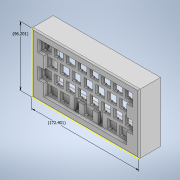
# Autodesk Inventor part: 1by2
Saved by Autodesk Inventor 2021 (Build 250183000, 183)
## iProperties
Created: 2021-06-14
Part Number: 1by2
Material: Generic
Document SubType Name: Modeling
Designer: UpahU
Density: 1 g/cm^3
Appearance: Default
Author: UpahU
Autodesk Inventor part; units mm, degrees
ref_plane "YZ Plane" through (0, 0, 0) normal (1, 0, 0) x (0, 1, 0)
ref_plane "XZ Plane" through (0, 0, 0) normal (0, 1, 0) x (-1, 0, 0)
ref_plane "XY Plane" through (0, 0, 0) normal (0, 0, 1) x (1, 0, 0)
sketch "Sketch1" plane through (0, 0, 0) normal (0, 0, 1) x (1, 0, 0)
  line L0 (0.0951, 96.5659) -> (172.496, 96.5659)
  line L1 (172.496, 96.5659) -> (172.496, 0.3652)
  line L2 (172.496, 0.3652) -> (0.0951, 0.3652)
  line L3 (0.0951, 0.3652) -> (0.0951, 96.5659)
  line L4 (136.445, 26.8911) -> (150.445, 26.8911)
  line L5 (150.445, 26.8911) -> (150.445, 12.8916)
  line L6 (150.445, 12.8916) -> (136.445, 12.8916)
  line L7 (136.445, 12.8916) -> (136.445, 26.8911)
  line L8 (117.394, 26.8911) -> (131.393, 26.8911)
  line L9 (131.3935, 26.8906) -> (131.393, 12.8911)
  line L10 (131.393, 12.8916) -> (117.394, 12.8916)
  line L11 (117.394, 12.8916) -> (117.394, 26.8911)
  line L12 (41.1939, 26.8911) -> (55.1931, 26.8911)
  line L13 (55.1931, 26.8911) -> (55.1931, 12.8916)
  line L14 (55.1931, 12.8916) -> (41.1939, 12.8916)
  line L15 (41.1939, 12.8916) -> (41.1939, 26.8911)
  line L16 (22.1437, 26.8911) -> (36.1446, 26.8911)
  line L17 (36.1446, 26.8911) -> (36.1446, 12.8916)
  line L18 (36.1446, 12.8916) -> (22.1437, 12.8916)
  line L19 (22.1437, 12.8916) -> (22.1437, 26.8911)
  line L20 (145.97, 45.9412) -> (159.97, 45.9412)
  line L21 (159.97, 45.9412) -> (159.97, 31.9416)
  line L22 (159.97, 31.9416) -> (145.97, 31.9416)
  line L23 (145.97, 31.9416) -> (145.97, 45.9412)
  line L24 (126.92, 45.9412) -> (140.92, 45.9412)
  line L25 (140.92, 45.9412) -> (140.92, 31.9416)
  line L26 (140.92, 31.9416) -> (126.92, 31.9416)
  line L27 (126.92, 31.9416) -> (126.92, 45.9412)
  line L28 (107.869, 45.9412) -> (121.868, 45.9412)
  line L29 (121.868, 45.9412) -> (121.868, 31.9416)
  line L30 (121.868, 31.9416) -> (107.869, 31.9416)
  line L31 (107.869, 31.9416) -> (107.869, 45.9412)
  line L32 (88.8199, 45.9412) -> (102.82, 45.9412)
  line L33 (102.82, 45.9412) -> (102.82, 31.9416)
  line L34 (102.82, 31.9416) -> (88.8199, 31.9416)
  line L35 (88.8199, 31.9416) -> (88.8199, 45.9412)
  line L36 (69.7699, 45.9412) -> (83.7696, 45.9412)
  line L37 (83.7696, 45.9412) -> (83.7696, 31.9416)
  line L38 (83.7696, 31.9416) -> (69.7699, 31.9416)
  line L39 (69.7699, 31.9416) -> (69.7699, 45.9412)
  line L40 (50.7199, 45.9412) -> (64.7196, 45.9412)
  line L41 (64.7196, 45.9412) -> (64.7196, 31.9416)
  line L42 (64.7196, 31.9416) -> (50.7199, 31.9416)
  line L43 (50.7199, 31.9416) -> (50.7199, 45.9412)
  line L44 (31.6701, 45.9412) -> (45.6696, 45.9412)
  line L45 (45.6696, 45.9412) -> (45.6696, 31.9416)
  line L46 (45.6696, 31.9416) -> (31.6701, 31.9416)
  line L47 (31.6701, 31.9416) -> (31.6701, 45.9412)
  line L48 (12.6201, 45.9412) -> (26.6196, 45.9412)
  line L49 (26.6196, 45.9412) -> (26.6196, 31.9416)
  line L50 (26.6196, 31.9416) -> (12.6201, 31.9416)
  line L51 (12.6201, 31.9416) -> (12.6201, 45.9412)
  line L52 (136.445, 64.9912) -> (150.445, 64.9912)
  line L53 (150.445, 64.9912) -> (150.445, 50.9916)
  line L54 (150.445, 50.9916) -> (136.445, 50.9916)
  line L55 (136.445, 50.9916) -> (136.445, 64.9912)
  line L56 (117.394, 64.9912) -> (131.393, 64.9912)
  line L57 (131.393, 64.9912) -> (131.393, 50.9916)
  line L58 (131.393, 50.9916) -> (117.394, 50.9916)
  line L59 (117.394, 50.9916) -> (117.394, 64.9912)
  line L60 (98.3439, 64.9912) -> (112.343, 64.9912)
  line L61 (112.343, 64.9912) -> (112.343, 50.9916)
  line L62 (112.343, 50.9916) -> (98.3439, 50.9916)
  line L63 (98.3439, 50.9916) -> (98.3439, 64.9912)
  line L64 (79.2939, 64.9912) -> (93.2931, 64.9912)
  line L65 (93.2931, 64.9912) -> (93.2931, 50.9916)
  line L66 (93.2931, 50.9916) -> (79.2939, 50.9916)
  line L67 (79.2939, 50.9916) -> (79.2939, 64.9912)
  line L68 (60.2439, 64.9912) -> (74.2431, 64.9912)
  line L69 (74.2431, 64.9912) -> (74.2431, 50.9916)
  line L70 (74.2431, 50.9916) -> (60.2439, 50.9916)
  line L71 (60.2439, 50.9916) -> (60.2439, 64.9912)
  line L72 (41.1939, 64.9912) -> (55.1931, 64.9912)
  line L73 (55.1931, 64.9912) -> (55.1931, 50.9916)
  line L74 (55.1931, 50.9916) -> (41.1939, 50.9916)
  line L75 (41.1939, 50.9916) -> (41.1939, 64.9912)
  line L76 (22.1437, 64.9912) -> (36.1446, 64.9912)
  line L77 (36.1446, 64.9912) -> (36.1446, 50.9916)
  line L78 (36.1446, 50.9916) -> (22.1437, 50.9916)
  line L79 (22.1437, 50.9916) -> (22.1437, 64.9912)
  line L80 (145.97, 84.0412) -> (159.97, 84.0412)
  line L81 (159.97, 84.0412) -> (159.97, 70.0416)
  line L82 (159.97, 70.0416) -> (145.97, 70.0416)
  line L83 (145.97, 70.0416) -> (145.97, 84.0412)
  line L84 (126.92, 84.0412) -> (140.92, 84.0412)
  line L85 (140.92, 84.0412) -> (140.92, 70.0416)
  line L86 (140.92, 70.0416) -> (126.92, 70.0416)
  line L87 (126.92, 70.0416) -> (126.92, 84.0412)
  line L88 (107.869, 84.0412) -> (121.868, 84.0412)
  line L89 (121.868, 84.0412) -> (121.868, 70.0416)
  line L90 (121.868, 70.0416) -> (107.869, 70.0416)
  line L91 (107.869, 70.0416) -> (107.869, 84.0412)
  line L92 (88.8199, 84.0412) -> (102.82, 84.0412)
  line L93 (102.82, 84.0412) -> (102.82, 70.0416)
  line L94 (102.82, 70.0416) -> (88.8199, 70.0416)
  line L95 (88.8199, 70.0416) -> (88.8199, 84.0412)
  line L96 (69.7699, 84.0412) -> (83.7696, 84.0412)
  line L97 (83.7696, 84.0412) -> (83.7696, 70.0416)
  line L98 (83.7696, 70.0416) -> (69.7699, 70.0416)
  line L99 (69.7699, 70.0416) -> (69.7699, 84.0412)
  line L100 (50.7199, 84.0412) -> (64.7196, 84.0412)
  line L101 (64.7196, 84.0412) -> (64.7196, 70.0416)
  line L102 (64.7196, 70.0416) -> (50.7199, 70.0416)
  line L103 (50.7199, 70.0416) -> (50.7199, 84.0412)
  line L104 (31.6701, 84.0412) -> (45.6696, 84.0412)
  line L105 (45.6696, 84.0412) -> (45.6696, 70.0416)
  line L106 (45.6696, 70.0416) -> (31.6701, 70.0416)
  line L107 (31.6701, 70.0416) -> (31.6701, 84.0412)
  line L108 (12.6201, 84.0412) -> (26.6196, 84.0412)
  line L109 (26.6196, 84.0412) -> (26.6196, 70.0416)
  line L110 (26.6196, 70.0416) -> (12.6201, 70.0416)
  line L111 (12.6201, 70.0416) -> (12.6201, 84.0412)
  line L112 (79.2923, 12.8885) -> (93.2923, 12.8885)
  line L113 (79.2923, 26.6885) -> (79.2923, 12.8885)
  line L114 (93.2923, 12.8885) -> (93.2923, 26.6885)
  arc A0 (108.8423, 29.7885) -> (108.3423, 30.2885) centre (108.3423, 29.7885) ccw
  arc A1 (101.8423, 10.6385) -> (102.3423, 10.1385) centre (102.3423, 10.6385) ccw
  arc A2 (108.3423, 10.1385) -> (108.8423, 10.6385) centre (108.3423, 10.6385) ccw
  line L115 (108.3423, 30.2885) -> (104.8423, 30.2885)
  line L116 (104.8423, 30.2885) -> (102.3423, 30.2885)
  line L117 (102.3423, 10.1385) -> (108.3423, 10.1385)
  line L118 (101.8423, 26.6885) -> (101.8423, 10.6385)
  line L119 (108.8423, 10.6385) -> (108.8423, 29.7885)
  arc A3 (64.2423, 30.2885) -> (63.7423, 29.7885) centre (64.2423, 29.7885) ccw
  arc A4 (63.7423, 10.6385) -> (64.2423, 10.1385) centre (64.2423, 10.6385) ccw
  arc A5 (70.2423, 10.1385) -> (70.7423, 10.6385) centre (70.2423, 10.6385) ccw
  line L120 (70.2423, 30.2885) -> (67.7423, 30.2885)
  line L121 (67.7423, 30.2885) -> (64.2423, 30.2885)
  line L122 (64.2423, 10.1385) -> (70.2423, 10.1385)
  line L123 (63.7423, 29.7885) -> (63.7423, 10.6385)
  line L124 (70.7423, 10.6385) -> (70.7423, 26.6885)
  line L125 (102.3423, 30.2885) -> (70.2423, 30.2885)
  line L126 (70.7423, 26.6885) -> (79.2923, 26.6885)
  line L127 (93.2923, 26.6885) -> (101.8423, 26.6885)
  point P0 (0.0951, 0.3652)
  point P1 (172.496, 0.3652)
  point P2 (131.3935, 26.8911)
  point P3 (131.393, 12.8916)
  point P4 (70.7423, 10.6385)
  point P5 (70.2423, 10.1385)
  point P6 (64.2423, 10.1385)
  point P7 (63.7423, 10.6385)
  point P8 (63.7423, 29.7885)
  point P9 (64.2423, 30.2885)
  point P10 (108.3423, 30.2885)
  point P11 (108.8423, 29.7885)
  point P12 (108.8423, 10.6385)
  point P13 (108.3423, 10.1385)
  point P14 (102.3423, 10.1385)
  point P15 (101.8423, 10.6385)
  point P16 (86.2923, 19.8914)
  constraints: 256 end point, 12 point on circle, 6 centre point
extrude "Extrusion1" add sketch "Sketch1" along normal blind 1.5
sketch "Sketch2" plane through (0, 0, 1.5) normal (0, 0, 1) x (1, 0, 0)
  line L0 (0.0951, 96.5659) -> (172.496, 96.5659)
  line L1 (172.496, 96.5659) -> (172.496, 0.3652)
  line L2 (172.496, 0.3652) -> (0.0951, 0.3652)
  line L3 (0.0951, 0.3652) -> (0.0951, 96.5659)
  line L4 (10.0928, 86.5685) -> (10.0928, 67.5157)
  line L5 (10.0928, 67.5157) -> (19.6178, 67.5157)
  line L6 (19.6178, 67.5157) -> (19.6178, 48.4671)
  line L7 (19.6178, 48.4671) -> (10.0928, 48.4671)
  line L8 (10.0928, 48.4671) -> (10.0928, 29.4156)
  line L9 (10.0928, 29.4156) -> (19.6178, 29.4156)
  line L10 (19.6178, 29.4156) -> (19.6178, 10.3656)
  line L11 (19.6178, 10.3656) -> (152.97, 10.3656)
  line L12 (152.97, 10.3656) -> (152.97, 29.4156)
  line L13 (152.97, 29.4156) -> (162.495, 29.4156)
  line L14 (162.495, 29.4156) -> (162.495, 48.4671)
  line L15 (162.495, 48.4671) -> (152.97, 48.4671)
  line L16 (152.97, 48.4671) -> (152.97, 67.5157)
  line L17 (152.97, 67.5157) -> (162.495, 67.5157)
  line L18 (162.495, 67.5157) -> (162.495, 86.5685)
  line L19 (162.495, 86.5685) -> (10.0928, 86.5685)
  point P0 (0, 0)
  point P1 (0.0951, 0.3652)
  point P2 (172.496, 0.3652)
  constraints: 40 end point
extrude "Extrusion2" add sketch "Sketch2" along normal blind 5
sketch "Sketch3" plane through (0, 0, 0) normal (0, 0, -1) x (-1, 0, 0)
  line L0 (-81.2961, 86.5671) -> (-162.497, 86.5671)
  line L1 (-162.497, 86.5671) -> (-162.497, 10.3656)
  line L2 (-162.497, 10.3656) -> (-10.0961, 10.3656)
  line L3 (-10.0961, 10.3656) -> (-10.0961, 86.5671)
  line L4 (-10.0961, 86.5671) -> (-81.2961, 86.5671)
  line L5 (-81.2961, 96.5659) -> (-0.0951, 96.5659)
  line L6 (-0.0951, 96.5659) -> (-0.0951, 0.3652)
  line L7 (-0.0951, 0.3652) -> (-172.496, 0.3652)
  line L8 (-172.496, 0.3652) -> (-172.496, 96.5659)
  line L9 (-172.496, 96.5659) -> (-81.2961, 96.5659)
  point P0 (0, 0)
  point P1 (-0.0951, 96.5659)
  point P2 (-172.496, 96.5659)
  point P3 (-0.0951, 0.3652)
  point P4 (-162.497, 10.3656)
  constraints: 20 end point, 2 horizontal
extrude "Extrusion3" add sketch "Sketch3" along normal blind 28.55
fillet "Fillet1" radius 2 4 edges at (86.2955, 0.3652, 6.5) (172.496, 48.4655, 6.5) (86.2955, 96.5659, 6.5) (0.0951, 48.4655, 6.5)
sketch "Sketch4" plane through (0, 0, -28.55) normal (0, 0, -1) x (-1, 0, 0)
  line L0 (-2.0951, 2.3652) -> (-2.0951, 94.5659) projected
  line L1 (-170.496, 2.3652) -> (-2.0951, 2.3652)
  line L2 (-2.0951, 2.3652) -> (-2.0951, 94.5659)
  line L3 (-2.0951, 94.5659) -> (-170.496, 94.5659)
  line L4 (-170.496, 94.5659) -> (-170.496, 2.3652)
  line L5 (-172.496, 0.3652) -> (-172.496, 96.5659) projected
  line L6 (-172.496, 0.3652) -> (-0.0338, 0.3652)
  line L7 (-0.0338, 0.3652) -> (-0.0338, 96.5659)
  line L8 (-0.0338, 96.5659) -> (-172.496, 96.5659)
  line L9 (-172.496, 96.5659) -> (-172.496, 0.3652)
  point P0 (0, 0)
  point P1 (-2.0951, 2.3652)
  constraints: 16 end point, 4 parallel, 2 horizontal, 2 perpendicular
extrude "Extrusion4" cut sketch "Sketch4" against normal blind 0.5
sketch "Sketch5" plane through (0, 0, 0) normal (0, 0, -1) x (-1, 0, 0)
  line L0 (-162.497, 86.5671) -> (-162.497, 10.3656) projected
  line L1 (-63.8234, 10.3656) -> (-10.0961, 10.3656) projected
  line L2 (-10.0961, 10.3656) -> (-10.0961, 86.5671) projected
  line L3 (-10.0961, 86.5671) -> (-162.497, 86.5671) projected
  line L4 (-12.6201, 84.0412) -> (-26.6196, 84.0412) projected
  line L5 (-12.6201, 70.0416) -> (-12.6201, 84.0412) projected
  line L6 (-26.6196, 70.0416) -> (-12.6201, 70.0416) projected
  line L7 (-26.6196, 84.0412) -> (-26.6196, 70.0416) projected
  line L8 (-31.6701, 84.0412) -> (-45.6696, 84.0412) projected
  line L9 (-31.6701, 70.0416) -> (-31.6701, 84.0412) projected
  line L10 (-45.6696, 70.0416) -> (-31.6701, 70.0416) projected
  line L11 (-45.6696, 84.0412) -> (-45.6696, 70.0416) projected
  line L12 (-50.7199, 84.0412) -> (-64.7196, 84.0412) projected
  line L13 (-50.7199, 70.0416) -> (-50.7199, 84.0412) projected
  line L14 (-64.7196, 70.0416) -> (-50.7199, 70.0416) projected
  line L15 (-64.7196, 84.0412) -> (-64.7196, 70.0416) projected
  line L16 (-69.7699, 84.0412) -> (-83.7696, 84.0412) projected
  line L17 (-69.7699, 70.0416) -> (-69.7699, 84.0412) projected
  line L18 (-83.7696, 70.0416) -> (-69.7699, 70.0416) projected
  line L19 (-83.7696, 84.0412) -> (-83.7696, 70.0416) projected
  line L20 (-88.8199, 84.0412) -> (-102.82, 84.0412) projected
  line L21 (-88.8199, 70.0416) -> (-88.8199, 84.0412) projected
  line L22 (-102.82, 70.0416) -> (-88.8199, 70.0416) projected
  line L23 (-102.82, 84.0412) -> (-102.82, 70.0416) projected
  line L24 (-107.869, 84.0412) -> (-121.868, 84.0412) projected
  line L25 (-107.869, 70.0416) -> (-107.869, 84.0412) projected
  line L26 (-121.868, 70.0416) -> (-107.869, 70.0416) projected
  line L27 (-121.868, 84.0412) -> (-121.868, 70.0416) projected
  line L28 (-126.92, 84.0412) -> (-140.92, 84.0412) projected
  line L29 (-126.92, 70.0416) -> (-126.92, 84.0412) projected
  line L30 (-140.92, 70.0416) -> (-126.92, 70.0416) projected
  line L31 (-140.92, 84.0412) -> (-140.92, 70.0416) projected
  line L32 (-145.97, 84.0412) -> (-159.97, 84.0412) projected
  line L33 (-145.97, 70.0416) -> (-145.97, 84.0412) projected
  line L34 (-159.97, 70.0416) -> (-145.97, 70.0416) projected
  line L35 (-159.97, 84.0412) -> (-159.97, 70.0416) projected
  line L36 (-22.1437, 64.9912) -> (-36.1446, 64.9912) projected
  line L37 (-22.1437, 50.9916) -> (-22.1437, 64.9912) projected
  line L38 (-36.1446, 50.9916) -> (-22.1437, 50.9916) projected
  line L39 (-36.1446, 64.9912) -> (-36.1446, 50.9916) projected
  line L40 (-41.1939, 64.9912) -> (-55.1931, 64.9912) projected
  line L41 (-41.1939, 50.9916) -> (-41.1939, 64.9912) projected
  line L42 (-55.1931, 50.9916) -> (-41.1939, 50.9916) projected
  line L43 (-55.1931, 64.9912) -> (-55.1931, 50.9916) projected
  line L44 (-60.2439, 64.9912) -> (-74.2431, 64.9912) projected
  line L45 (-60.2439, 50.9916) -> (-60.2439, 64.9912) projected
  line L46 (-74.2431, 50.9916) -> (-60.2439, 50.9916) projected
  line L47 (-74.2431, 64.9912) -> (-74.2431, 50.9916) projected
  line L48 (-79.2939, 64.9912) -> (-93.2931, 64.9912) projected
  line L49 (-79.2939, 50.9916) -> (-79.2939, 64.9912) projected
  line L50 (-93.2931, 50.9916) -> (-79.2939, 50.9916) projected
  line L51 (-93.2931, 64.9912) -> (-93.2931, 50.9916) projected
  line L52 (-98.3439, 64.9912) -> (-112.343, 64.9912) projected
  line L53 (-98.3439, 50.9916) -> (-98.3439, 64.9912) projected
  line L54 (-112.343, 50.9916) -> (-98.3439, 50.9916) projected
  line L55 (-112.343, 64.9912) -> (-112.343, 50.9916) projected
  line L56 (-117.394, 64.9912) -> (-131.393, 64.9912) projected
  line L57 (-117.394, 50.9916) -> (-117.394, 64.9912) projected
  line L58 (-131.393, 50.9916) -> (-117.394, 50.9916) projected
  line L59 (-131.393, 64.9912) -> (-131.393, 50.9916) projected
  line L60 (-136.445, 64.9912) -> (-150.445, 64.9912) projected
  line L61 (-136.445, 50.9916) -> (-136.445, 64.9912) projected
  line L62 (-150.445, 50.9916) -> (-136.445, 50.9916) projected
  line L63 (-150.445, 64.9912) -> (-150.445, 50.9916) projected
  line L64 (-12.6201, 45.9412) -> (-26.6196, 45.9412) projected
  line L65 (-12.6201, 31.9416) -> (-12.6201, 45.9412) projected
  line L66 (-26.6196, 31.9416) -> (-12.6201, 31.9416) projected
  line L67 (-26.6196, 45.9412) -> (-26.6196, 31.9416) projected
  line L68 (-31.6701, 45.9412) -> (-45.6696, 45.9412) projected
  line L69 (-31.6701, 31.9416) -> (-31.6701, 45.9412) projected
  line L70 (-45.6696, 31.9416) -> (-31.6701, 31.9416) projected
  line L71 (-45.6696, 45.9412) -> (-45.6696, 31.9416) projected
  line L72 (-50.7199, 45.9412) -> (-64.7196, 45.9412) projected
  line L73 (-50.7199, 31.9416) -> (-50.7199, 45.9412) projected
  line L74 (-64.7196, 31.9416) -> (-50.7199, 31.9416) projected
  line L75 (-64.7196, 45.9412) -> (-64.7196, 31.9416) projected
  line L76 (-69.7699, 45.9412) -> (-83.7696, 45.9412) projected
  line L77 (-69.7699, 31.9416) -> (-69.7699, 45.9412) projected
  line L78 (-83.7696, 31.9416) -> (-69.7699, 31.9416) projected
  line L79 (-83.7696, 45.9412) -> (-83.7696, 31.9416) projected
  line L80 (-88.8199, 45.9412) -> (-102.82, 45.9412) projected
  line L81 (-88.8199, 31.9416) -> (-88.8199, 45.9412) projected
  line L82 (-102.82, 31.9416) -> (-88.8199, 31.9416) projected
  line L83 (-102.82, 45.9412) -> (-102.82, 31.9416) projected
  line L84 (-107.869, 45.9412) -> (-121.868, 45.9412) projected
  line L85 (-107.869, 31.9416) -> (-107.869, 45.9412) projected
  line L86 (-121.868, 31.9416) -> (-107.869, 31.9416) projected
  line L87 (-121.868, 45.9412) -> (-121.868, 31.9416) projected
  line L88 (-126.92, 45.9412) -> (-140.92, 45.9412) projected
  line L89 (-126.92, 31.9416) -> (-126.92, 45.9412) projected
  line L90 (-140.92, 31.9416) -> (-126.92, 31.9416) projected
  line L91 (-140.92, 45.9412) -> (-140.92, 31.9416) projected
  line L92 (-145.97, 45.9412) -> (-159.97, 45.9412) projected
  line L93 (-145.97, 31.9416) -> (-145.97, 45.9412) projected
  line L94 (-159.97, 31.9416) -> (-145.97, 31.9416) projected
  line L95 (-159.97, 45.9412) -> (-159.97, 31.9416) projected
  line L96 (-22.1437, 26.8911) -> (-36.1446, 26.8911) projected
  line L97 (-22.1437, 12.8916) -> (-22.1437, 26.8911) projected
  line L98 (-36.1446, 12.8916) -> (-22.1437, 12.8916) projected
  line L99 (-36.1446, 26.8911) -> (-36.1446, 12.8916) projected
  line L100 (-41.1939, 26.8911) -> (-55.1931, 26.8911) projected
  line L101 (-41.1939, 12.8916) -> (-41.1939, 26.8911) projected
  line L102 (-55.1931, 12.8916) -> (-41.1939, 12.8916) projected
  line L103 (-55.1931, 26.8911) -> (-55.1931, 12.8916) projected
  line L104 (-117.394, 26.8911) -> (-131.3935, 26.8911) projected
  line L105 (-117.394, 12.8916) -> (-117.394, 26.8911) projected
  line L106 (-131.393, 12.8916) -> (-117.394, 12.8916) projected
  line L107 (-131.3935, 26.8911) -> (-131.393, 12.8916) projected
  line L108 (-136.445, 26.8911) -> (-150.445, 26.8911) projected
  line L109 (-136.445, 12.8916) -> (-136.445, 26.8911) projected
  line L110 (-150.445, 12.8916) -> (-136.445, 12.8916) projected
  line L111 (-150.445, 26.8911) -> (-150.445, 12.8916) projected
  line L112 (-10.0961, 10.3656) -> (-10.0961, 86.5671) projected
  line L113 (-162.497, 86.5671) -> (-10.0961, 86.5671)
  line L114 (-10.0961, 86.5671) -> (-10.0961, 10.3656)
  line L115 (-10.0961, 10.3656) -> (-162.497, 10.3656)
  line L116 (-162.497, 10.3656) -> (-162.497, 86.5671)
  line L117 (-156.47, 85.0414) -> (-149.47, 85.0414)
  line L118 (-149.47, 85.0414) -> (-149.47, 69.0414)
  line L119 (-149.47, 69.0414) -> (-156.47, 69.0414)
  line L120 (-156.47, 69.0414) -> (-156.47, 85.0414)
  line L121 (-156.47, 85.0414) -> (-149.47, 69.0414) construction
  line L122 (-149.47, 85.0414) -> (-156.47, 69.0414) construction
  line L123 (-137.42, 85.0414) -> (-130.42, 85.0414)
  line L124 (-130.42, 85.0414) -> (-130.42, 69.0414)
  line L125 (-130.42, 69.0414) -> (-137.42, 69.0414)
  line L126 (-137.42, 69.0414) -> (-137.42, 85.0414)
  line L127 (-137.42, 85.0414) -> (-130.42, 69.0414) construction
  line L128 (-130.42, 85.0414) -> (-137.42, 69.0414) construction
  line L129 (-118.3685, 85.0414) -> (-111.3685, 85.0414)
  line L130 (-111.3685, 85.0414) -> (-111.3685, 69.0414)
  line L131 (-111.3685, 69.0414) -> (-118.3685, 69.0414)
  line L132 (-118.3685, 69.0414) -> (-118.3685, 85.0414)
  line L133 (-118.3685, 85.0414) -> (-111.3685, 69.0414) construction
  line L134 (-111.3685, 85.0414) -> (-118.3685, 69.0414) construction
  line L135 (-99.3199, 85.0414) -> (-92.3199, 85.0414)
  line L136 (-92.3199, 85.0414) -> (-92.3199, 69.0414)
  line L137 (-92.3199, 69.0414) -> (-99.3199, 69.0414)
  line L138 (-99.3199, 69.0414) -> (-99.3199, 85.0414)
  line L139 (-99.3199, 85.0414) -> (-92.3199, 69.0414) construction
  line L140 (-92.3199, 85.0414) -> (-99.3199, 69.0414) construction
  line L141 (-80.2698, 85.0414) -> (-73.2698, 85.0414)
  line L142 (-73.2698, 85.0414) -> (-73.2698, 69.0414)
  line L143 (-73.2698, 69.0414) -> (-80.2698, 69.0414)
  line L144 (-80.2698, 69.0414) -> (-80.2698, 85.0414)
  line L145 (-80.2698, 85.0414) -> (-73.2698, 69.0414) construction
  line L146 (-73.2698, 85.0414) -> (-80.2698, 69.0414) construction
  line L147 (-61.2197, 85.0414) -> (-54.2198, 85.0414)
  line L148 (-54.2198, 85.0414) -> (-54.2198, 69.0414)
  line L149 (-54.2198, 69.0414) -> (-61.2197, 69.0414)
  line L150 (-61.2197, 69.0414) -> (-61.2197, 85.0414)
  line L151 (-61.2197, 85.0414) -> (-54.2198, 69.0414) construction
  line L152 (-54.2198, 85.0414) -> (-61.2197, 69.0414) construction
  line L153 (-42.1699, 85.0414) -> (-35.1699, 85.0414)
  line L154 (-35.1699, 85.0414) -> (-35.1699, 69.0414)
  line L155 (-35.1699, 69.0414) -> (-42.1699, 69.0414)
  line L156 (-42.1699, 69.0414) -> (-42.1699, 85.0414)
  line L157 (-42.1699, 85.0414) -> (-35.1699, 69.0414) construction
  line L158 (-35.1699, 85.0414) -> (-42.1699, 69.0414) construction
  line L159 (-23.1198, 85.0414) -> (-16.1198, 85.0414)
  line L160 (-16.1198, 85.0414) -> (-16.1198, 69.0414)
  line L161 (-16.1198, 69.0414) -> (-23.1198, 69.0414)
  line L162 (-23.1198, 69.0414) -> (-23.1198, 85.0414)
  line L163 (-23.1198, 85.0414) -> (-16.1198, 69.0414) construction
  line L164 (-16.1198, 85.0414) -> (-23.1198, 69.0414) construction
  line L165 (-32.6442, 65.9914) -> (-25.6441, 65.9914)
  line L166 (-25.6441, 65.9914) -> (-25.6441, 49.9914)
  line L167 (-25.6441, 49.9914) -> (-32.6442, 49.9914)
  line L168 (-32.6442, 49.9914) -> (-32.6442, 65.9914)
  line L169 (-32.6442, 65.9914) -> (-25.6441, 49.9914) construction
  line L170 (-25.6441, 65.9914) -> (-32.6442, 49.9914) construction
  line L171 (-51.6935, 49.9914) -> (-44.6935, 49.9914)
  line L172 (-44.6935, 49.9914) -> (-44.6935, 65.9914)
  line L173 (-44.6935, 65.9914) -> (-51.6935, 65.9914)
  line L174 (-51.6935, 65.9914) -> (-51.6935, 49.9914)
  line L175 (-51.6935, 49.9914) -> (-44.6935, 65.9914) construction
  line L176 (-44.6935, 49.9914) -> (-51.6935, 65.9914) construction
  line L177 (-70.7435, 49.9914) -> (-63.7435, 49.9914)
  line L178 (-63.7435, 49.9914) -> (-63.7435, 65.9914)
  line L179 (-63.7435, 65.9914) -> (-70.7435, 65.9914)
  line L180 (-70.7435, 65.9914) -> (-70.7435, 49.9914)
  line L181 (-70.7435, 49.9914) -> (-63.7435, 65.9914) construction
  line L182 (-63.7435, 49.9914) -> (-70.7435, 65.9914) construction
  line L183 (-89.7965, 49.9914) -> (-82.7965, 49.9914)
  line L184 (-82.7965, 49.9914) -> (-82.7965, 65.9914)
  line L185 (-82.7965, 65.9914) -> (-89.7965, 65.9914)
  line L186 (-89.7965, 65.9914) -> (-89.7965, 49.9914)
  line L187 (-89.7965, 49.9914) -> (-82.7965, 65.9914) construction
  line L188 (-82.7965, 49.9914) -> (-89.7965, 65.9914) construction
  line L189 (-108.8445, 49.9914) -> (-101.8445, 49.9914)
  line L190 (-101.8445, 49.9914) -> (-101.8445, 65.9914)
  line L191 (-101.8445, 65.9914) -> (-108.8445, 65.9914)
  line L192 (-108.8445, 65.9914) -> (-108.8445, 49.9914)
  line L193 (-108.8445, 49.9914) -> (-101.8445, 65.9914) construction
  line L194 (-101.8445, 49.9914) -> (-108.8445, 65.9914) construction
  line L195 (-127.8935, 49.9914) -> (-120.8935, 49.9914)
  line L196 (-120.8935, 49.9914) -> (-120.8935, 65.9914)
  line L197 (-120.8935, 65.9914) -> (-127.8935, 65.9914)
  line L198 (-127.8935, 65.9914) -> (-127.8935, 49.9914)
  line L199 (-127.8935, 49.9914) -> (-120.8935, 65.9914) construction
  line L200 (-120.8935, 49.9914) -> (-127.8935, 65.9914) construction
  line L201 (-146.945, 49.9914) -> (-139.945, 49.9914)
  line L202 (-139.945, 49.9914) -> (-139.945, 65.9914)
  line L203 (-139.945, 65.9914) -> (-146.945, 65.9914)
  line L204 (-146.945, 65.9914) -> (-146.945, 49.9914)
  line L205 (-146.945, 49.9914) -> (-139.945, 65.9914) construction
  line L206 (-139.945, 49.9914) -> (-146.945, 65.9914) construction
  line L207 (-156.47, 30.9414) -> (-149.47, 30.9414)
  line L208 (-149.47, 30.9414) -> (-149.47, 46.9414)
  line L209 (-149.47, 46.9414) -> (-156.47, 46.9414)
  line L210 (-156.47, 46.9414) -> (-156.47, 30.9414)
  line L211 (-156.47, 30.9414) -> (-149.47, 46.9414) construction
  line L212 (-149.47, 30.9414) -> (-156.47, 46.9414) construction
  line L213 (-137.42, 46.9414) -> (-130.42, 46.9414)
  line L214 (-130.42, 46.9414) -> (-130.42, 30.9414)
  line L215 (-130.42, 30.9414) -> (-137.42, 30.9414)
  line L216 (-137.42, 30.9414) -> (-137.42, 46.9414)
  line L217 (-137.42, 46.9414) -> (-130.42, 30.9414) construction
  line L218 (-130.42, 46.9414) -> (-137.42, 30.9414) construction
  line L219 (-118.3685, 46.9414) -> (-111.3685, 46.9414)
  line L220 (-111.3685, 46.9414) -> (-111.3685, 30.9414)
  line L221 (-111.3685, 30.9414) -> (-118.3685, 30.9414)
  line L222 (-118.3685, 30.9414) -> (-118.3685, 46.9414)
  line L223 (-118.3685, 46.9414) -> (-111.3685, 30.9414) construction
  line L224 (-111.3685, 46.9414) -> (-118.3685, 30.9414) construction
  line L225 (-99.3199, 46.9414) -> (-92.3199, 46.9414)
  line L226 (-92.3199, 46.9414) -> (-92.3199, 30.9414)
  line L227 (-92.3199, 30.9414) -> (-99.3199, 30.9414)
  line L228 (-99.3199, 30.9414) -> (-99.3199, 46.9414)
  line L229 (-99.3199, 46.9414) -> (-92.3199, 30.9414) construction
  line L230 (-92.3199, 46.9414) -> (-99.3199, 30.9414) construction
  line L231 (-80.2698, 46.9414) -> (-73.2698, 46.9414)
  line L232 (-73.2698, 46.9414) -> (-73.2698, 30.9414)
  line L233 (-73.2698, 30.9414) -> (-80.2698, 30.9414)
  line L234 (-80.2698, 30.9414) -> (-80.2698, 46.9414)
  line L235 (-80.2698, 46.9414) -> (-73.2698, 30.9414) construction
  line L236 (-73.2698, 46.9414) -> (-80.2698, 30.9414) construction
  line L237 (-61.2197, 46.9414) -> (-54.2198, 46.9414)
  line L238 (-54.2198, 46.9414) -> (-54.2198, 30.9414)
  line L239 (-54.2198, 30.9414) -> (-61.2197, 30.9414)
  line L240 (-61.2197, 30.9414) -> (-61.2197, 46.9414)
  line L241 (-61.2197, 46.9414) -> (-54.2198, 30.9414) construction
  line L242 (-54.2198, 46.9414) -> (-61.2197, 30.9414) construction
  line L243 (-42.1699, 46.9414) -> (-35.1699, 46.9414)
  line L244 (-35.1699, 46.9414) -> (-35.1699, 30.9414)
  line L245 (-35.1699, 30.9414) -> (-42.1699, 30.9414)
  line L246 (-42.1699, 30.9414) -> (-42.1699, 46.9414)
  line L247 (-42.1699, 46.9414) -> (-35.1699, 30.9414) construction
  line L248 (-35.1699, 46.9414) -> (-42.1699, 30.9414) construction
  line L249 (-23.1198, 46.9414) -> (-16.1198, 46.9414)
  line L250 (-16.1198, 46.9414) -> (-16.1198, 30.9414)
  line L251 (-16.1198, 30.9414) -> (-23.1198, 30.9414)
  line L252 (-23.1198, 30.9414) -> (-23.1198, 46.9414)
  line L253 (-23.1198, 46.9414) -> (-16.1198, 30.9414) construction
  line L254 (-16.1198, 46.9414) -> (-23.1198, 30.9414) construction
  line L255 (-32.6442, 11.8914) -> (-25.6441, 11.8914)
  line L256 (-25.6441, 11.8914) -> (-25.6441, 27.8913)
  line L257 (-25.6441, 27.8913) -> (-32.6442, 27.8913)
  line L258 (-32.6442, 27.8913) -> (-32.6442, 11.8914)
  line L259 (-32.6442, 11.8914) -> (-25.6441, 27.8913) construction
  line L260 (-25.6441, 11.8914) -> (-32.6442, 27.8913) construction
  line L261 (-51.6935, 11.8914) -> (-44.6935, 11.8914)
  line L262 (-44.6935, 11.8914) -> (-44.6935, 27.8913)
  line L263 (-44.6935, 27.8913) -> (-51.6935, 27.8913)
  line L264 (-51.6935, 27.8913) -> (-51.6935, 11.8914)
  line L265 (-51.6935, 11.8914) -> (-44.6935, 27.8913) construction
  line L266 (-44.6935, 11.8914) -> (-51.6935, 27.8913) construction
  line L267 (-89.7965, 11.8914) -> (-82.7965, 11.8914)
  line L268 (-82.7965, 11.8914) -> (-82.7965, 27.8913)
  line L269 (-82.7965, 27.8913) -> (-89.7965, 27.8913)
  line L270 (-89.7965, 27.8913) -> (-89.7965, 11.8914)
  line L271 (-89.7965, 11.8914) -> (-82.7965, 27.8913) construction
  line L272 (-82.7965, 11.8914) -> (-89.7965, 27.8913) construction
  line L273 (-127.8935, 11.8914) -> (-120.8935, 11.8914)
  line L274 (-120.8935, 11.8914) -> (-120.8935, 27.8913)
  line L275 (-120.8935, 27.8913) -> (-127.8935, 27.8913)
  line L276 (-127.8935, 27.8913) -> (-127.8935, 11.8914)
  line L277 (-127.8935, 11.8914) -> (-120.8935, 27.8913) construction
  line L278 (-120.8935, 11.8914) -> (-127.8935, 27.8913) construction
  line L279 (-146.945, 11.8914) -> (-139.945, 11.8914)
  line L280 (-139.945, 11.8914) -> (-139.945, 27.8913)
  line L281 (-139.945, 27.8913) -> (-146.945, 27.8913)
  line L282 (-146.945, 27.8913) -> (-146.945, 11.8914)
  line L283 (-146.945, 11.8914) -> (-139.945, 27.8913) construction
  line L284 (-139.945, 11.8914) -> (-146.945, 27.8913) construction
  line L285 (-63.8681, 9.1218) -> (-108.7191, 9.1218)
  line L286 (-19.6178, 10.3656) -> (-152.97, 10.3656) projected
  line L287 (-101.968, 25.4208) -> (-108.7191, 25.4208) projected
  line L288 (-152.97, 10.3656) -> (-19.6178, 10.3656) projected
  line L289 (-63.8681, 25.4208) -> (-63.8681, 10.3656)
  line L290 (-63.8681, 10.3656) -> (-108.7191, 10.3656)
  line L291 (-108.7191, 10.3656) -> (-108.7191, 25.4208)
  line L292 (-108.7191, 25.4208) -> (-101.968, 25.4208)
  line L293 (-101.968, 25.4208) -> (-101.968, 27.8913)
  line L294 (-101.968, 27.8913) -> (-108.7191, 27.8913)
  line L295 (-108.7191, 27.8913) -> (-108.7191, 25.4208)
  line L296 (-63.8681, 25.4208) -> (-70.6191, 25.4208) projected
  line L297 (-63.8681, 25.4208) -> (-70.6191, 25.4208)
  line L298 (-70.6191, 25.4208) -> (-70.6191, 27.8913)
  line L299 (-70.6191, 27.8913) -> (-63.8681, 27.8913)
  line L300 (-63.8681, 27.8913) -> (-63.8681, 25.4208)
  line L301 (-63.7423, 10.6385) -> (-63.7423, 29.7885) projected
  arc A0 (-63.8234, 10.3656) -> (-63.7423, 10.6385) centre (-64.2423, 10.6385) ccw projected
  arc A1 (-70.7423, 10.6385) -> (-70.6613, 10.3656) centre (-70.2423, 10.6385) ccw projected
  line L302 (-70.7423, 26.6885) -> (-70.7423, 10.6385) projected
  line L303 (-79.2923, 26.6885) -> (-70.7423, 26.6885) projected
  line L304 (-79.2923, 12.8885) -> (-79.2923, 26.6885) projected
  line L305 (-93.2923, 12.8885) -> (-79.2923, 12.8885) projected
  line L306 (-93.2923, 26.6885) -> (-93.2923, 12.8885) projected
  line L307 (-101.8423, 26.6885) -> (-93.2923, 26.6885) projected
  line L308 (-101.8423, 10.6385) -> (-101.8423, 26.6885) projected
  arc A2 (-101.9234, 10.3656) -> (-101.8423, 10.6385) centre (-102.3423, 10.6385) ccw projected
  arc A3 (-108.8423, 10.6385) -> (-108.7613, 10.3656) centre (-108.3423, 10.6385) ccw projected
  line L309 (-108.8423, 29.7885) -> (-108.8423, 10.6385) projected
  line L310 (-101.9234, 10.3656) -> (-70.6613, 10.3656) projected
  line L311 (-162.497, 10.3656) -> (-108.7613, 10.3656) projected
  arc A4 (-108.3423, 30.2885) -> (-108.8423, 29.7885) centre (-108.3423, 29.7885) ccw projected
  line L312 (-64.2423, 30.2885) -> (-108.3423, 30.2885) projected
  arc A5 (-63.7423, 29.7885) -> (-64.2423, 30.2885) centre (-64.2423, 29.7885) ccw projected
  point P0 (0, 0)
  point P1 (-152.97, 77.0414)
  point P2 (-133.92, 77.0414)
  point P3 (-114.8685, 77.0414)
  point P4 (-95.8199, 77.0414)
  point P5 (-76.7698, 77.0414)
  point P6 (-57.7198, 77.0414)
  point P7 (-38.6699, 77.0414)
  point P8 (-19.6198, 77.0414)
  point P9 (-143.445, 57.9914)
  point P10 (-124.3935, 57.9914)
  point P11 (-86.2965, 57.9914)
  point P12 (-48.1935, 57.9914)
  point P13 (-29.1441, 57.9914)
  point P14 (-67.2435, 57.9914)
  point P15 (-105.3445, 57.9914)
  point P16 (-152.97, 38.9414)
  point P17 (-133.92, 38.9414)
  point P18 (-114.8685, 38.9414)
  point P19 (-95.8199, 38.9414)
  point P20 (-76.7698, 38.9414)
  point P21 (-57.7198, 38.9414)
  point P22 (-38.6699, 38.9414)
  point P23 (-19.6198, 38.9414)
  point P24 (-86.2965, 19.8914)
  point P25 (-143.445, 19.8914)
  point P26 (-124.3935, 19.8914)
  point P27 (-48.1935, 19.8914)
  point P28 (-29.1441, 19.8914)
  point P29 (-44.6935, 50.9916)
  point P30 (-51.6935, 50.9916)
  point P31 (-51.6935, 64.9912)
  point P32 (-44.6935, 64.9912)
  point P33 (-63.7435, 50.9916)
  point P34 (-70.7435, 50.9916)
  point P35 (-70.7435, 64.9912)
  point P36 (-63.7435, 64.9912)
  point P37 (-82.7965, 50.9916)
  point P38 (-89.7965, 50.9916)
  point P39 (-89.7965, 64.9912)
  point P40 (-82.7965, 64.9912)
  point P41 (-101.8445, 50.9916)
  point P42 (-108.8445, 50.9916)
  point P43 (-108.8445, 64.9912)
  point P44 (-101.8445, 64.9912)
  point P45 (-120.8935, 50.9916)
  point P46 (-127.8935, 50.9916)
  point P47 (-127.8935, 64.9912)
  point P48 (-120.8935, 64.9912)
  point P49 (-139.945, 50.9916)
  point P50 (-146.945, 50.9916)
  point P51 (-146.945, 64.9912)
  point P52 (-139.945, 64.9912)
  point P53 (-149.47, 31.9416)
  point P54 (-156.47, 31.9416)
  point P55 (-156.47, 45.9412)
  point P56 (-149.47, 45.9412)
  point P57 (-25.6441, 12.8916)
  point P58 (-32.6442, 12.8916)
  point P59 (-32.6442, 26.8911)
  point P60 (-25.6441, 26.8911)
  point P61 (-44.6935, 12.8916)
  point P62 (-51.6935, 12.8916)
  point P63 (-51.6935, 26.8911)
  point P64 (-44.6935, 26.8911)
  point P65 (-120.8935, 12.8916)
  point P66 (-127.8935, 12.8916)
  point P67 (-127.8935, 26.8911)
  point P68 (-120.8935, 26.8911)
  point P69 (-139.945, 12.8916)
  point P70 (-146.945, 12.8916)
  point P71 (-146.945, 26.8911)
  point P72 (-139.945, 26.8911)
  point P73 (-16.1198, 31.9416)
  point P74 (-23.1198, 31.9416)
  point P75 (-23.1198, 45.9412)
  point P76 (-16.1198, 45.9412)
  point P77 (-35.1699, 31.9416)
  point P78 (-42.1699, 31.9416)
  point P79 (-42.1699, 45.9412)
  point P80 (-35.1699, 45.9412)
  point P81 (-54.2198, 31.9416)
  point P82 (-61.2197, 31.9416)
  point P83 (-61.2197, 45.9412)
  point P84 (-54.2198, 45.9412)
  point P85 (-73.2698, 31.9416)
  point P86 (-80.2698, 31.9416)
  point P87 (-80.2698, 45.9412)
  point P88 (-73.2698, 45.9412)
  point P89 (-92.3199, 31.9416)
  point P90 (-99.3199, 31.9416)
  point P91 (-99.3199, 45.9412)
  point P92 (-92.3199, 45.9412)
  point P93 (-111.3685, 31.9416)
  point P94 (-118.3685, 31.9416)
  point P95 (-118.3685, 45.9412)
  point P96 (-111.3685, 45.9412)
  point P97 (-130.42, 31.9416)
  point P98 (-137.42, 31.9416)
  point P99 (-137.42, 45.9412)
  point P100 (-130.42, 45.9412)
  point P101 (-25.6441, 50.9916)
  point P102 (-32.6442, 50.9916)
  point P103 (-32.6442, 64.9912)
  point P104 (-25.6441, 64.9912)
  point P105 (-16.1198, 70.0416)
  point P106 (-23.1198, 70.0416)
  point P107 (-23.1198, 84.0412)
  point P108 (-16.1198, 84.0412)
  point P109 (-35.1699, 70.0416)
  point P110 (-42.1699, 70.0416)
  point P111 (-42.1699, 84.0412)
  point P112 (-35.1699, 84.0412)
  point P113 (-54.2198, 70.0416)
  point P114 (-61.2197, 70.0416)
  point P115 (-61.2197, 84.0412)
  point P116 (-54.2198, 84.0412)
  point P117 (-73.2698, 70.0416)
  point P118 (-80.2698, 70.0416)
  point P119 (-80.2698, 84.0412)
  point P120 (-73.2698, 84.0412)
  point P121 (-92.3199, 70.0416)
  point P122 (-99.3199, 70.0416)
  point P123 (-99.3199, 84.0412)
  point P124 (-92.3199, 84.0412)
  point P125 (-111.3685, 70.0416)
  point P126 (-118.3685, 70.0416)
  point P127 (-118.3685, 84.0412)
  point P128 (-111.3685, 84.0412)
  point P129 (-130.42, 70.0416)
  point P130 (-137.42, 70.0416)
  point P131 (-137.42, 84.0412)
  point P132 (-130.42, 84.0412)
  point P133 (-149.47, 70.0416)
  point P134 (-156.47, 70.0416)
  point P135 (-156.47, 84.0412)
  point P136 (-149.47, 84.0412)
  point P137 (-108.7191, 19.3918)
  point P138 (-108.7191, 13.1218)
  point P139 (-109.5432, 19.3918)
  point P140 (-108.7191, 22.1906)
  point P141 (-101.968, 22.1906)
  point P142 (-93.2932, 22.1906)
  point P143 (-79.2939, 26.8911)
  point P144 (-79.2939, 22.1906)
  point P145 (-70.6191, 22.1906)
  point P146 (-63.8681, 22.1906)
  point P147 (-63.044, 22.1906)
  point P148 (-109.5432, 22.1906)
  point P149 (-63.044, 19.3918)
  point P150 (-108.8423, 10.3656)
  point P151 (-63.7423, 10.3656)
  point P152 (-63.8234, 10.3656)
  point P153 (-101.9234, 10.3656)
  point P154 (-70.6613, 10.3656)
  point P155 (-101.9234, 10.3656)
  point P156 (-70.6613, 10.3656)
  point P157 (-89.7965, 12.8885)
  point P158 (-82.7965, 12.8885)
  dimension "d9" = 7
  dimension "d10" = 16
  dimension "d11" = 7
  dimension "d12" = 16
  dimension "d13" = 7
  dimension "d14" = 16
  dimension "d15" = 7
  dimension "d16" = 16
  dimension "d17" = 7
  dimension "d18" = 7
  dimension "d19" = 7
  dimension "d20" = 7
  dimension "d21" = 7
  dimension "d22" = 16
  dimension "d23" = 7
  dimension "d24" = 7
  dimension "d25" = 16
  dimension "d26" = 7
  dimension "d27" = 16
  dimension "d28" = 7
  dimension "d29" = 16
  dimension "d30" = 7
  dimension "d31" = 7
  dimension "d32" = 16
  dimension "d33" = 7
  dimension "d34" = 16
  dimension "d35" = 7
  dimension "d36" = 16
  dimension "d37" = 7
  dimension "d38" = 16
  dimension "d39" = 7
  dimension "d40" = 16
  dimension "d41" = 7
  dimension "d42" = 16
  dimension "d43" = 7
  dimension "d44" = 16
  dimension "d45" = 7
  dimension "d46" = 16
  dimension "d47" = 7
  dimension "d48" = 16
  dimension "d49" = 7
  dimension "d50" = 16
  dimension "d51" = 7
  dimension "d52" = 16
  dimension "d53" = 7
  dimension "d54" = 16
  dimension "d55" = 7
  dimension "d56" = 16
  dimension "d57" = 7
  dimension "d58" = 16
  constraints: 368 end point, 63 parallel, 56 midpoint, 31 horizontal, 31 perpendicular, 7 point on line
  measures "d9" distance of L118.end L119.end
  measures "d10" distance of L117.end L118.end
  measures "d11" distance of L124.end L125.end
  measures "d12" distance of L123.end L124.end
  measures "d13" distance of L130.end L131.end
  measures "d14" distance of L129.end L130.end
  measures "d15" distance of L136.end L137.end
  measures "d16" distance of L135.end L136.end
  measures "d17" distance of L142.end L143.end
  measures "d18" distance of L148.end L149.end
  measures "d19" distance of L154.end L155.end
  measures "d20" distance of L160.end L161.end
  measures "d21" distance of L166.end L167.end
  measures "d22" distance of L165.end L166.end
  measures "d23" distance of L173.end L172.end
  measures "d24" distance of L179.end L178.end
  measures "d25" distance of L178.end L177.end
  measures "d26" distance of L185.end L184.end
  measures "d27" distance of L184.end L183.end
  measures "d28" distance of L191.end L190.end
  measures "d29" distance of L190.end L189.end
  measures "d30" distance of L197.end L196.end
  measures "d31" distance of L203.end L202.end
  measures "d32" distance of L202.end L201.end
  measures "d33" distance of L209.end L208.end
  measures "d34" distance of L208.end L207.end
  measures "d35" distance of L214.end L215.end
  measures "d36" distance of L213.end L214.end
  measures "d37" distance of L220.end L221.end
  measures "d38" distance of L219.end L220.end
  measures "d39" distance of L226.end L227.end
  measures "d40" distance of L225.end L226.end
  measures "d41" distance of L232.end L233.end
  measures "d42" distance of L231.end L232.end
  measures "d43" distance of L238.end L239.end
  measures "d44" distance of L237.end L238.end
  measures "d45" distance of L244.end L245.end
  measures "d46" distance of L243.end L244.end
  measures "d47" distance of L250.end L251.end
  measures "d48" distance of L249.end L250.end
  measures "d49" distance of L257.end L256.end
  measures "d50" distance of L256.end L255.end
  measures "d51" distance of L263.end L262.end
  measures "d52" distance of L262.end L261.end
  measures "d53" distance of L269.end L268.end
  measures "d54" distance of L268.end L267.end
  measures "d55" distance of L275.end L274.end
  measures "d56" distance of L274.end L273.end
  measures "d57" distance of L281.end L280.end
  measures "d58" distance of L280.end L279.end
extrude "Extrusion5" add sketch "Sketch5" along normal blind 3 contours L3 L2 L1 A0 L301 A5 L312 A4 L309 A3 L115 L0 | A2 L308 L307 L306 L305 L270 L267 L268 L304 L303 L302 A1 L115
sketch "Sketch6" plane through (0.0951, 0.3652, 4.5) normal (-1, 0, 0) x (0, 0, 1)
  line L0 (-7.5, 69.6764) -> (-3, 69.6764) projected
  line L1 (-7.5, 83.676) -> (-3, 83.676) projected
  line L2 (-7.5, 69.6764) -> (-7.5, 83.676) projected
  line L3 (-9, 80.676) -> (-13, 80.676)
  line L4 (-13, 80.676) -> (-13, 72.676)
  line L5 (-13, 72.676) -> (-9, 72.676)
  line L6 (-9, 72.676) -> (-9, 80.676)
  line L7 (-3, 83.676) -> (-3, 69.6764) projected
  point P0 (-4.5, -0.3652)
  dimension "d62" = 4
  dimension "d63" = 8
  dimension "d64" = 3
  dimension "d79" = 10
  constraints: 8 end point, 2 parallel, 1 horizontal, 1 perpendicular
  measures "d62" distance of L3.start L3.end
  measures "d63" distance of L3.end L4.end
  measures "d64" distance between parallel lines of L3 L1
  measures "d79" distance between parallel lines of L7 L4
extrude "Extrusion6" cut sketch "Sketch6" against normal up to next contours L6 L5 L4 L3
sketch "Sketch7" plane through (0.0951, 0.3652, 4.5) normal (-1, 0, 0) x (0, 0, 1)
  line L0 (-9, 72.676) -> (-13, 72.676) projected
  line L1 (-13, 72.676) -> (-13, 80.676) projected
  line L2 (-13, 80.676) -> (-9, 80.676) projected
  line L3 (-9, 80.676) -> (-9, 72.676) projected
  line L4 (-32.55, 96.2007) -> (-32.55, 0) projected
  line L5 (0, 0) -> (-32.55, 0) projected
  line L6 (0, 96.2007) -> (0, 0) projected
  line L7 (-32.55, 96.2007) -> (0, 96.2007) projected
  line L8 (-7, 83.676) -> (-15, 83.676)
  line L9 (-15, 83.676) -> (-15, 69.676)
  line L10 (-15, 69.676) -> (-7, 69.676)
  line L11 (-7, 69.676) -> (-7, 83.676)
  point P0 (-4.5, -0.3652)
  dimension "d67" = 3
  dimension "d68" = 3
  dimension "d69" = 2
  dimension "d70" = 2
  constraints: 8 end point, 2 parallel, 1 horizontal, 1 perpendicular
  measures "d67" distance between parallel lines of L8 L2
  measures "d68" distance between parallel lines of L10 L0
  measures "d69" distance between parallel lines of L11 L3
  measures "d70" distance between parallel lines of L9 L1
extrude "Extrusion7" cut sketch "Sketch7" against normal blind 8 contours L11 L10 L9 L8
chamfer "Chamfer1" distance 2 angle 45 4 edges at (8.0951, 77.0412, -4.5) (8.0951, 81.0412, -6.5) (8.0951, 77.0412, -8.5) (8.0951, 73.0412, -6.5)
sketch "Sketch9" plane through (0, 0, 1.5) normal (0, 0, 1) x (1, 0, 0)
  point P0 (0, 0)
extrude "Extrusion8" [suppressed]
sketch "Sketch11" plane through (10.0961, 10.3656, -28.55) normal (1, 0, 0) x (0, 0, -1)
  line L0 (-19.05, 56.1756) -> (-18.05, 56.1756)
  line L1 (-18.05, 56.1756) -> (-18.05, 76.1756)
  line L2 (-18.05, 76.1756) -> (-19.05, 76.1756)
  line L3 (-19.05, 76.1756) -> (-19.05, 56.1756)
  line L4 (-30.05, 76.2029) -> (-30.05, 57.1501) projected
  line L5 (-24.05, 62.6756) -> (-20.05, 62.6756) projected
  line L6 (-19.05, 56.1756) -> (-25, 56.1756)
  line L7 (-25, 56.1756) -> (-25, 57.1756)
  line L8 (-25, 57.1756) -> (-19.05, 57.1756)
  line L9 (-19.05, 57.1756) -> (-19.05, 56.1756)
  point P0 (-28.55, -10.3656)
  dimension "d80" = 11
  dimension "d81" = 20
  dimension "d82" = 6.5
  dimension "d83" = 1
  dimension "d84" = 1
  constraints: 16 end point, 4 parallel, 2 horizontal, 2 perpendicular
  measures "d80" distance between parallel lines of L3 L4
  measures "d81" distance of L0.end L1.end
  measures "d82" distance between parallel lines of L5 L0
  measures "d83" distance of L0.start L0.end
  measures "d84" distance of L6.end L7.end
extrude "Extrusion9" add sketch "Sketch11" along normal blind 1.5
sketch "Sketch15" plane through (0, 0, 6.5) normal (0, 0, 1) x (1, 0, 0)
  line L0 (0.0951, 96.5659) -> (0.0951, 0.3652) projected
  line L1 (0.0951, 0.3652) -> (172.496, 0.3652) projected
  point P0 (0, 0)
  dimension "d91" = 96.2007
  dimension "d92" = 172.4009
  measures "d91" distance of L0.start L0.end
  measures "d92" distance of L0.end L1.end
sketch "Sketch16" plane through (0.0951, 0.3652, 4.5) normal (0, -1, 0) x (1, 0, 0)
  point P0 (-0.0951, -4.5)
sketch "Sketch17" plane through (0, 0, -3) normal (0, 0, -1) x (-1, 0, 0)
  line L0 (-89.7965, 27.8913) -> (-82.7965, 27.8913) projected
  line L1 (-10.0961, 10.3656) -> (-162.497, 10.3656) projected
  line L2 (-108.7191, 22.1906) -> (-108.7191, 25.4208) projected
  line L3 (-63.8681, 25.4208) -> (-63.8681, 22.1906) projected
  line L4 (-101.968, 17.5907) -> (-101.968, 13.1218) projected
  line L5 (-70.6191, 13.1218) -> (-70.6191, 17.5907) projected
  line L6 (-10.0961, 10.3656) -> (-162.497, 10.3656) projected
  line L7 (-108.7191, 27.8913) -> (-101.968, 27.8913)
  line L8 (-101.968, 27.8913) -> (-101.968, 10.3656)
  line L9 (-101.968, 10.3656) -> (-108.7191, 10.3656)
  line L10 (-108.7191, 10.3656) -> (-108.7191, 27.8913)
  line L11 (-63.8681, 27.8913) -> (-70.6191, 27.8913)
  line L12 (-70.6191, 27.8913) -> (-70.6191, 10.3656)
  line L13 (-70.6191, 10.3656) -> (-63.8681, 10.3656)
  line L14 (-63.8681, 10.3656) -> (-63.8681, 27.8913)
  line L15 (-109.5432, 19.3918) -> (-108.7191, 19.3918) projected
  line L16 (-108.7191, 19.3918) -> (-63.8681, 19.3918)
  line L17 (-63.8681, 19.3918) -> (-63.8681, 10.3656)
  line L18 (-63.8681, 10.3656) -> (-108.7191, 10.3656)
  line L19 (-108.7191, 10.3656) -> (-108.7191, 19.3918)
  point P0 (0, 0)
  point P1 (-70.6191, 19.3918)
  point P2 (-101.968, 19.3918)
  constraints: 24 end point, 6 parallel, 3 horizontal, 3 perpendicular, 3 point on line
extrude "Extrusion10" [suppressed]
equation "\"d68\" = d67"
equation "\"d70\" = d69"
body "Solid1"
